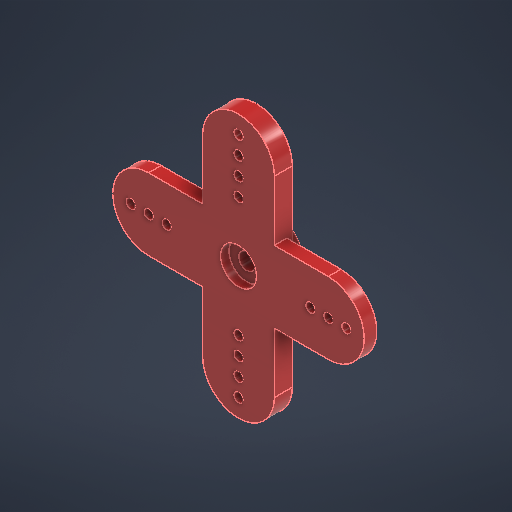
# Autodesk Inventor part: Servo Horn 3 Skiba
Saved by Autodesk Inventor 2027.1 (Build 311270010, 270A)
## iProperties
Created: 2020-09-11
Part Number: Servo Horn 3 Skiba
Material: Generic
Document SubType Name: Modeling
Designer: 239tr
Density: 1 g/cm^3
Appearance: Red
Mass: 2.2251 g
Surface Area: 23.5214 cm^2
Volume: 2.2251 cm^3
Author: 239tr
Autodesk Inventor part; units mm, degrees
ref_plane "YZ Plane" through (0, 0, 0) normal (1, 0, 0) x (0, 1, 0)
ref_plane "XZ Plane" through (0, 0, 0) normal (0, 1, 0) x (-1, 0, 0)
ref_plane "XY Plane" through (0, 0, 0) normal (0, 0, 1) x (1, 0, 0)
sketch "Sketch1" plane through (0, 0, 0) normal (0, 0, 1) x (1, 0, 0)
  arc A0 (6, 16) -> (-6, 16) centre (0, 16) ccw
  line L0 (0, -30.8) -> (0, 30.8) construction
  line L1 (-6, 16) -> (-6, 6)
  line L2 (6, 16) -> (6, 6)
  circle A1 centre (0, 13) radius 0.75
  circle A2 centre (0, 10) radius 0.75
  circle A3 centre (0, 19) radius 0.75
  circle A4 centre (0, 16) radius 0.75
  line L3 (-7.8151, 0) -> (8.8196, 0) construction
  arc A5 (-6, -16) -> (6, -16) centre (0, -16) ccw
  line L4 (-6, -16) -> (-6, -6)
  line L5 (6, -16) -> (6, -6)
  circle A6 centre (0, -13) radius 0.75
  circle A7 centre (0, -10) radius 0.75
  circle A8 centre (0, -19) radius 0.75
  circle A9 centre (0, -16) radius 0.75
  line L6 (6, 6) -> (15, 6)
  arc A10 (15, -6) -> (15, 6) centre (15, 0) ccw
  line L7 (15, 6) -> (15, -6) construction
  line L8 (15, 6) -> (27, 6) construction
  line L9 (15, -6) -> (6, -6)
  circle A11 centre (18, 0) radius 0.75
  circle A12 centre (15, 0) radius 0.75
  circle A13 centre (12, 0) radius 0.75
  line L10 (7.8151, 0) -> (-8.8196, 0) construction
  line L11 (-6, 6) -> (-15, 6)
  arc A14 (-15, 6) -> (-15, -6) centre (-15, 0) ccw
  line L12 (-15, 6) -> (-15, -6) construction
  line L13 (-15, -6) -> (-6, -6)
  circle A15 centre (-18, 0) radius 0.75
  circle A16 centre (-15, 0) radius 0.75
  circle A17 centre (-12, 0) radius 0.75
  line L14 (6, 6) -> (6, -6)
  line L15 (-6, 6) -> (-6, -6)
  point P0 (0, 0)
  dimension "d0" = 12
  dimension "d1" = 6
  dimension "d2" = 10
  dimension "d3" = 10
  dimension "d5" = 1.5
  dimension "d6" = 1.5
  dimension "d8" = 1.5
  dimension "d9" = 13
  dimension "d10" = 10
  dimension "d11" = 19
  dimension "d12" = 1.5
  dimension "d13" = 16
  dimension "d14" = 16
  dimension "d15" = 10
  dimension "d16" = 90
  dimension "d17" = 6
  dimension "d18" = 15
  dimension "d19" = 12
  dimension "d20" = 15
  dimension "d21" = 18
  dimension "d22" = 1.5
  dimension "d23" = 1.5
  dimension "d24" = 1.5
  dimension "d25" = 6
  dimension "d26" = 6
  constraints: 30 end point, 18 centre point, 17 symmetric about line, 8 point on circle, 7 point on line, 4 horizontal, 3 vertical, 1 parallel, 1 perpendicular, 1 tangent, 9 other
  measures "d0" distance of L1.start L2.start
  measures "d1" radius of A0
  measures "d2" distance of L1.start L1.end
  measures "d3" distance of L2.start L2.end
  measures "d5" diameter of A1
  measures "d6" diameter of A2
  measures "d8" diameter of A3
  measures "d9" distance of point (0, 0) A1.centre
  measures "d10" distance of point (0, 0) A2.centre
  measures "d11" distance of point (0, 0) A3.centre
  measures "d12" diameter of A4
  measures "d13" distance of point (0, 0) A4.centre
  measures "d14" distance of point (0, 0) A0.centre
  measures "d15" distance of A7.centre point (0, 0)
  measures "d16" angle of L7 L8
  measures "d17" radius of A10
  measures "d18" distance of A10.centre point (0, 0)
  measures "d19" distance of point (0, 0) A13.centre
  measures "d20" distance of point (0, 0) A12.centre
  measures "d21" distance of A11.centre point (0, 0)
  measures "d22" diameter of A13
  measures "d23" diameter of A12
  measures "d24" diameter of A11
  measures "d25" distance from line of L6 A12.centre
  measures "d26" distance from line of L6 A11.centre
extrude "Extrusion1" add sketch "Sketch1" against normal blind 3 contours L2 L14 L5 A5 L4 L15 L1 A0
extrude "Extrusion2" add sketch "Sketch1" against normal blind 2.1 contours L6 A10 L9 L14 | L15 L13 A14 L11
sketch "Sketch2" plane through (0, 0, -3) normal (0, 0, -1) x (-1, 0, 0)
  circle A0 centre (0, 0) radius 5
  dimension "d31" = 10
  constraints: 1 centre point, 1 coincident
  measures "d31" diameter of A0
extrude "Extrusion3" add sketch "Sketch2" along normal blind 2.85
sketch "Sketch3" plane through (0, 0, -5.85) normal (0, 0, -1) x (-1, 0, 0)
  point P0 (0, 0)
  point P1 (0, 0)
  constraints: 1 coincident
hole "Hole1" at (0, 0, -5.85) direction (0, 0, 1) diameter 5.5 depth 2.85
sketch "Sketch6" plane through (0, 0, 0) normal (0, 0, 1) x (1, 0, 0)
  point P0 (0, 0)
  point P1 (0, 0)
  constraints: 1 coincident
hole "Hole2" at (0, 0, 0) direction (0, 0, -1) diameter 6 depth 1.4
sketch "Sketch7" plane through (0, 0, -1.4) normal (0, 0, 1) x (1, 0, 0)
  point P0 (0, 0)
  point P1 (0, 0)
  constraints: 1 coincident
hole "Hole3" at (0, 0, -1.4) direction (0, 0, -1) diameter 2.7 end through all
equation "\"d2\" = d3"
equation "\"d5\" = d8"
equation "\"d6\" = d8"
equation "\"d12\" = d8"
equation "\"d15\" = d10"
equation "\"d22\" = d8"
equation "\"d23\" = d8"
equation "\"d24\" = d8"
body "Solid1"
